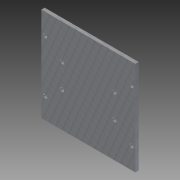
# Autodesk Inventor part: xy axis mount
Saved by Autodesk Inventor 2011 (Build 150239000, 239)
## iProperties
Created: 2013-10-30
Part Number: xy axis mount
Document SubType Name: Modeling
Designer: Devon
Density: 1 g/cm^3
Author: Devon
Autodesk Inventor part; units mm, degrees
ref_plane "YZ Plane" through (0, 0, 0) normal (1, 0, 0) x (0, 1, 0)
ref_plane "XZ Plane" through (0, 0, 0) normal (0, 1, 0) x (-1, 0, 0)
ref_plane "XY Plane" through (0, 0, 0) normal (0, 0, 1) x (1, 0, 0)
sketch "Sketch1" plane through (0, 0, 0) normal (0, 0, 1) x (1, 0, 0)
  line L0 (-68.9114, 68.2476) -> (111.0984, 68.2476)
  line L1 (111.0984, 68.2476) -> (111.0984, -111.7622)
  line L2 (111.0984, -111.7622) -> (-68.9114, -111.7622)
  line L3 (-68.9114, -111.7622) -> (-68.9114, 68.2476)
  line L4 (111.0984, 68.2476) -> (111.0984, 28.2426)
  line L5 (-68.9114, 68.2476) -> (-61.4184, 68.2476)
  line L6 (111.0984, 68.2476) -> (103.6054, 68.2476)
  line L7 (111.0984, -111.7622) -> (111.0984, -71.7572)
  circle A0 centre (-61.4184, 28.2426) radius 3.81
  circle A1 centre (-61.4184, -71.7572) radius 3.81
  circle A2 centre (103.6054, -71.7572) radius 3.81
  circle A3 centre (103.6054, 28.2426) radius 3.81
  circle A4 centre (71.1061, 1.2551) radius 3.81
  circle A5 centre (-28.9191, 1.2551) radius 3.81
  circle A6 centre (-28.9191, -44.7697) radius 3.81
  circle A7 centre (71.1061, -44.7697) radius 3.81
  point P0 (0, 0)
  dimension "d0" = 180.0098
  dimension "d1" = 180.0098
  dimension "d2" = 40.005
  dimension "d3" = 7.493
  dimension "d4" = 7.493
  dimension "d5" = 40.005
  dimension "d10" = 7.62
  dimension "d11" = 7.62
  dimension "d12" = 7.62
  dimension "d13" = 7.62
  dimension "d14" = 7.62
  dimension "d15" = 7.62
  dimension "d16" = 7.62
  dimension "d17" = 7.62
  constraints: 16 end point, 8 centre point, 4 point on line, 2 parallel, 1 horizontal, 1 perpendicular
  measures "d0" distance of L1.end L2.end
  measures "d1" distance of L0.end L1.end
  measures "d2" distance of L0.end L4.end
  measures "d3" distance of L0.start L5.end
  measures "d4" distance of L0.end L6.end
  measures "d5" distance of L1.end L7.end
  measures "d10" diameter of A0
  measures "d11" diameter of A1
  measures "d12" diameter of A2
  measures "d13" diameter of A3
  measures "d14" diameter of A4
  measures "d15" diameter of A5
  measures "d16" diameter of A6
  measures "d17" diameter of A7
extrude "Extrusion1" add sketch "Sketch1" along normal blind 6.35
body "Solid1"
